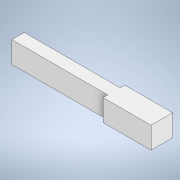
# Autodesk Inventor part: Key--D
Saved by Autodesk Inventor 2021 (Build 250183000, 183)
## iProperties
Created: 2021-03-17
Part Number: Key--D
Material: Generic
Document SubType Name: Modeling
Designer: Tom
Density: 1 g/cm^3
Appearance: White
Author: Tom
Autodesk Inventor part; units mm, degrees
ref_plane "YZ Plane" through (0, 0, 0) normal (1, 0, 0) x (0, 1, 0)
ref_plane "XZ Plane" through (0, 0, 0) normal (0, 1, 0) x (-1, 0, 0)
ref_plane "XY Plane" through (0, 0, 0) normal (0, 0, 1) x (1, 0, 0)
sketch "Sketch1" plane through (0, 0, 0) normal (0, 1, 0) x (-1, 0, 0)
  line L0 (0, 0) -> (49.2125, 0)
  line L1 (49.2125, 0) -> (49.2125, -4.7625)
  line L2 (49.2125, -4.7625) -> (147.6375, -4.7625)
  line L3 (147.6375, -4.7625) -> (147.6375, -17.4625)
  line L4 (147.6375, -17.4625) -> (49.2125, -17.4625)
  line L5 (49.2125, -17.4625) -> (49.2125, -22.225)
  line L6 (49.2125, -22.225) -> (0, -22.225)
  line L7 (0, -22.225) -> (0, 0)
  dimension "d0" = 22.225
  dimension "d1" = 147.6375
  dimension "d2" = 98.425
  dimension "d4" = 17.4625
  dimension "d5" = 17.4625
  constraints: 16 end point, 6 perpendicular, 2 point on line, 1 horizontal
  measures "d0" distance of L6.end L0.start
  measures "d1" horizontal distance of L2.end L0.start
  measures "d2" distance of L3.end L4.end
  measures "d4" distance from line of L0 L4.end
  measures "d5" distance from line of L1.end L6
extrude "Extrusion1" add sketch "Sketch1" against normal blind 22.225
body "Solid1"
